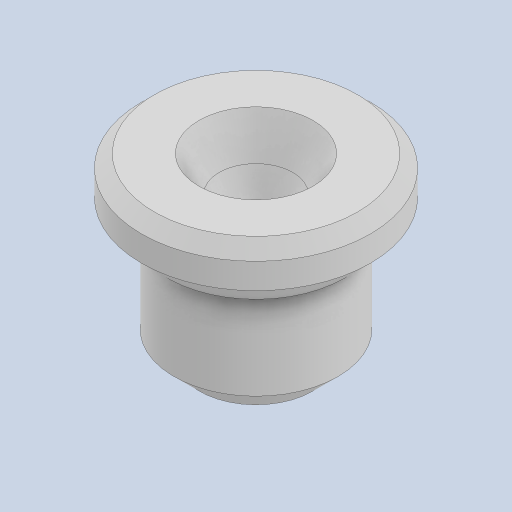
# Autodesk Inventor part: drop_funnel_v2
Saved by Autodesk Inventor 2024 (Build 280153000, 153)
## iProperties
Created: 2022-05-09
Part Number: drop_funnel_v2
Material: Generic
Document SubType Name: Modeling
Designer: to172
Density: 1 g/cm^3
Appearance: Default
Author: to172
Autodesk Inventor part; units mm, degrees
ref_plane "YZ Plane" through (0, 0, 0) normal (1, 0, 0) x (0, 1, 0)
ref_plane "XZ Plane" through (0, 0, 0) normal (0, 1, 0) x (-1, 0, 0)
ref_plane "XY Plane" through (0, 0, 0) normal (0, 0, 1) x (1, 0, 0)
sketch "Sketch1" plane through (0, 0, 0) normal (0, 0, 1) x (1, 0, 0)
  line L0 (0, 0) -> (0, 5.2441) construction
  line L1 (0, 0) -> (4.3793, 0) construction
  line L2 (2.9035, 11.25) -> (4.4912, 14)
  line L3 (0.425, 0) -> (0.425, 0.4889) construction
  line L4 (0.425, 0) -> (6.45, 0)
  line L5 (6.45, 0) -> (6.45, 9)
  line L6 (6.45, 9) -> (9, 9)
  line L7 (9, 9) -> (9, 14)
  line L8 (9, 14) -> (4.4912, 14)
  line L9 (0.425, 0) -> (0.425, 2)
  arc A0 (2.9035, 11.25) -> (0.425, 2) centre (18.925, 2) ccw
  dimension "d0" = 0.425
  dimension "d1" = 30
  dimension "d2" = 6.45
  dimension "d3" = 9
  dimension "d4" = 5
  dimension "d6" = 9
  dimension "d14" = 2
  dimension "d15" = 18.5
  constraints: 21 end point, 3 perpendicular, 3 point on line, 2 point on circle, 2 tangent, 2 vertical, 1 centre point, 1 horizontal, 1 parallel
  measures "d0" distance between parallel lines of L3 L0
  measures "d1" angle of L2 L0
  measures "d2" distance between parallel lines of L0 L5
  measures "d3" distance between parallel lines of L6 L1
  measures "d4" distance between parallel lines of L8 L6
  measures "d6" distance between parallel lines of L0 L7
  measures "d14" distance of L3.start L9.end
  measures "d15" radius of A0
revolve "Revolution1" add sketch "Sketch1" angle 360 about axis through (0, 0, 0) along (0, 1, 0)
chamfer "Chamfer1" distance 2 angle 45 1 edges at (-9, 9, 0)
chamfer "Chamfer2" distance 2 angle 45 1 edges at (-6.45, 0, 0)
chamfer "Chamfer3" distance 0.5 angle 45 1 edges at (-0.425, 0, 0)
chamfer "Chamfer4" distance 1 angle 45 1 edges at (-9, 14, 0)
body "Solid1"
